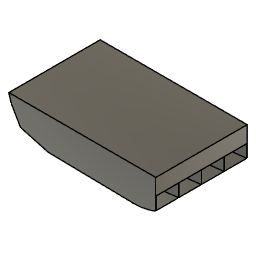
Downey-X-43A_scram_jet v2 (Autodesk Fusion 360 design; units mm, degrees)
Autodesk Fusion 360 part; units mm, degrees
sketch "Sketch12" plane through (0, 0, 0) normal (0, 1, 0) x (1, 0, 0)
  line L0 (2462.784, 249.936) -> (2462.784, 73.152)
  line L1 (2462.784, 73.152) -> (1681.0044, 73.152)
  line L2 (1681.0044, 73.152) -> (1700.784, 140.208)
  line L3 (1700.784, 140.208) -> (1749.552, 225.552)
  line L4 (1749.552, 225.552) -> (1894.3719, 265.9217)
  line L5 (1894.3719, 265.9217) -> (2340.864, 274.32)
  spline S0 degree 5 poles (2340.864, 274.32) (2342.4398, 274.4034) (2345.6372, 274.5328) (2350.5712, 274.6154) (2357.4276, 274.5004) (2366.4636, 273.9737) (2375.9522, 273.0575) (2385.8496, 271.7528) (2396.0651, 270.0751) (2406.4407, 268.0637) (2416.7336, 265.7899) (2426.6497, 263.3444) (2435.8739, 260.8263) (2444.1011, 258.3322) (2451.0699, 255.9464) (2456.5986, 253.7294) (2459.8206, 252.1119) (2461.5627, 250.9891) (2462.4265, 250.2804) (2462.784, 249.936) knots 0 0 0 0 0 0 0.066667 0.133333 0.2 0.266667 0.333333 0.4 0.466667 0.533333 0.6 0.666667 0.733333 0.8 0.866667 0.933333 1 1 1 1 1 1
  point P0 (2395.3801, 270.1209)
  point P1 (2450.592, 256.032)
  constraint vertical L0
  constraint perpendicular L0 L1
extrude "Extrude9" add sketch "Sketch12" along normal blind 853.44
sketch "Sketch13" plane through (0, 0, 0) normal (1, 0, 0) x (0, 1, 0)
  line L0 (883.92, -60.96) -> (-30.48, -60.96)
  line L1 (-30.48, -60.96) -> (-30.48, -304.8)
  line L2 (-30.48, -304.8) -> (883.92, -304.8)
  line L3 (883.92, -304.8) -> (883.92, -60.96)
  line L4 (713.232, -97.536) -> (231.648, -97.536)
  line L5 (231.648, -97.536) -> (231.648, -274.32)
  line L6 (231.648, -274.32) -> (713.232, -274.32)
  line L7 (713.232, -274.32) -> (713.232, -97.536)
  constraint horizontal L0
  constraint vertical L1
  constraint horizontal L2
  constraint vertical L3
  constraint horizontal L4
  constraint vertical L5
  constraint horizontal L6
  constraint vertical L7
extrude "Extrude10" cut sketch "Sketch13" along normal blind 3992.88
sketch "Sketch14" plane through (0, 0, 0) normal (1, 0, 0) x (0, 1, 0)
  line L0 (682.752, -201.168) -> (621.792, -201.168)
  line L1 (621.792, -201.168) -> (621.792, -231.648)
  line L2 (621.792, -231.648) -> (682.752, -231.648)
  line L3 (682.752, -231.648) -> (682.752, -201.168)
  line L4 (562.8742, -201.168) -> (501.9142, -201.168)
  line L5 (501.9142, -201.168) -> (501.9142, -231.648)
  line L6 (501.9142, -231.648) -> (562.8742, -231.648)
  line L7 (562.8742, -231.648) -> (562.8742, -201.168)
  line L8 (442.9963, -201.168) -> (382.0363, -201.168)
  line L9 (382.0363, -201.168) -> (382.0363, -231.648)
  line L10 (382.0363, -231.648) -> (442.9963, -231.648)
  line L11 (442.9963, -231.648) -> (442.9963, -201.168)
  line L12 (323.1185, -201.168) -> (262.1585, -201.168)
  line L13 (262.1585, -201.168) -> (262.1585, -231.648)
  line L14 (262.1585, -231.648) -> (323.1185, -231.648)
  line L15 (323.1185, -231.648) -> (323.1185, -201.168)
  line L16 (231.648, -97.536) -> (231.648, -249.936)
  line L17 (713.232, -140.208) -> (713.232, -225.552)
  dimension "d29" = 60.96
  dimension "d30" = 30.48
  dimension "d33" = -119.8778
  dimension "d34" = 0
  dimension "d44" = 30.48
  constraint horizontal L0
  constraint vertical L1
  constraint horizontal L2
  constraint vertical L3
  measures "d29" distance of L0.start L0.end
  measures "d30" distance of L0.start L2.end
  measures "d44" distance of L3 L17
extrude "Extrude11" cut sketch "Sketch14" along normal blind 4572
chamfer "Chamfer1" distance 36.576 distance2 286.512 4 edges at (1735.6183, 652.272, -201.168) (1735.6183, 532.3942, -201.168) (1735.6183, 412.5163, -201.168) (1735.6183, 292.6385, -201.168) measured on face at (1712.3954, 482.2647, -160.528) measured on face at (1712.3954, 482.2647, -160.528) measured on face at (1712.3954, 482.2647, -160.528) measured on face at (1712.3954, 482.2647, -160.528)
chamfer "Chamfer2" distance 24.384 distance2 121.92 8 edges at (1733.5118, 682.752, -197.4816) (1733.5118, 621.792, -197.4816) (1733.5118, 562.8742, -197.4816) (1733.5118, 501.9142, -197.4816) (1733.5118, 442.9963, -197.4816) (1733.5118, 382.0363, -197.4816) (1733.5118, 323.1185, -197.4816) (1733.5118, 262.1585, -197.4816) measured on face at (1738.8585, 602.1527, -206.8384) measured on face at (1738.8585, 602.1527, -206.8384) measured on face at (1738.8585, 602.1527, -206.8384) measured on face at (1738.8585, 602.1527, -206.8384) measured on face at (1738.8585, 602.1527, -206.8384) measured on face at (1738.8585, 602.1527, -206.8384) measured on face at (1738.8585, 602.1527, -206.8384) measured on face at (1738.8585, 602.1527, -206.8384)
chamfer "Chamfer4" distance 18.288 distance2 60.96 8 edges at (2462.784, 292.6385, -231.648) (2462.784, 412.5163, -231.648) (2462.784, 532.3942, -231.648) (2462.784, 652.272, -231.648) (2462.784, 652.272, -201.168) (2462.784, 532.3942, -201.168) (2462.784, 412.5163, -201.168) (2462.784, 292.6385, -201.168) measured on face at (2462.784, 462.6254, -132.08) measured on face at (2462.784, 462.6254, -132.08) measured on face at (2462.784, 462.6254, -132.08) measured on face at (2462.784, 462.6254, -132.08) measured on face at (2462.784, 462.6254, -132.08) measured on face at (2462.784, 462.6254, -132.08) measured on face at (2462.784, 462.6254, -132.08) measured on face at (2462.784, 462.6254, -132.08)
chamfer "Chamfer5" distance 28.3464 distance2 60.96 8 edges at (2462.784, 323.1185, -216.408) (2462.784, 382.0363, -216.408) (2462.784, 442.9963, -216.408) (2462.784, 501.9142, -216.408) (2462.784, 562.8742, -216.408) (2462.784, 621.792, -216.408) (2462.784, 682.752, -216.408) (2462.784, 262.1585, -216.408) measured on face at (2462.784, 462.6254, -125.984) measured on face at (2462.784, 462.6254, -125.984) measured on face at (2462.784, 462.6254, -125.984) measured on face at (2462.784, 462.6254, -125.984) measured on face at (2462.784, 462.6254, -125.984) measured on face at (2462.784, 462.6254, -125.984) measured on face at (2462.784, 462.6254, -125.984) measured on face at (2462.784, 462.6254, -125.984)
